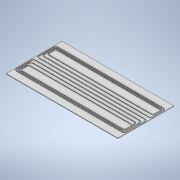
# Autodesk Inventor part: wire_holder_lasercutting800
Saved by Autodesk Inventor 2021 (Build 250183000, 183)
## iProperties
Created: 2021-02-03
Part Number: wire_holder_lasercutting800
Material: Generic
Document SubType Name: Modeling
Designer: User
Density: 1 g/cm^3
Appearance: Default
Author: User
Autodesk Inventor part; units mm, degrees
ref_plane "YZ Plane" through (0, 0, 0) normal (1, 0, 0) x (0, 1, 0)
ref_plane "XZ Plane" through (0, 0, 0) normal (0, 1, 0) x (-1, 0, 0)
ref_plane "XY Plane" through (0, 0, 0) normal (0, 0, 1) x (1, 0, 0)
sketch "Sketch1" plane through (0, 0, 0) normal (0, 1, 0) x (-1, 0, 0)
  line L0 (-18.4221, -16) -> (-503.4221, -16)
  line L1 (-518.4221, -1) -> (-518.4221, 135)
  line L2 (-503.4221, 150) -> (256.5779, 150)
  line L3 (271.5779, 135) -> (271.5779, 26)
  line L4 (-18.4221, -11) -> (-503.4221, -11)
  line L5 (-513.4221, -1) -> (-513.4221, 135)
  line L6 (-503.4221, 145) -> (256.5779, 145)
  line L7 (266.5779, 135) -> (266.5779, 26)
  line L8 (256.5779, 16) -> (-493.4221, 16)
  line L9 (-503.4221, 26) -> (-503.4221, 125)
  line L10 (256.5779, 11) -> (-493.4221, 11)
  line L11 (-508.4221, 26) -> (-508.4221, 125)
  line L12 (-493.4221, 135) -> (246.5779, 135)
  line L13 (-493.4221, 140) -> (246.5779, 140)
  line L14 (256.5779, 125) -> (256.5779, 53)
  line L15 (246.5779, 43) -> (-483.4221, 43)
  line L16 (261.5779, 125) -> (261.5779, 53)
  line L17 (246.5779, 38) -> (-483.4221, 38)
  line L18 (-493.4221, 53) -> (-493.4221, 115)
  line L19 (-483.4221, 125) -> (236.5779, 125)
  line L20 (246.5779, 115) -> (246.5779, 80)
  line L21 (236.5779, 70) -> (-488.4221, 70)
  line L22 (-498.4221, 53) -> (-498.4221, 115)
  line L23 (-483.4221, 130) -> (236.5779, 130)
  line L24 (251.5779, 115) -> (251.5779, 80)
  line L25 (236.5779, 65) -> (-488.4221, 65)
  line L26 (-488.4221, 70) -> (-488.4221, 65)
  line L27 (-123.4221, 150) -> (-123.4221, -150) construction
  line L28 (-18.4221, -11) -> (256.5779, -11)
  line L29 (271.5779, -26) -> (271.5779, -135)
  line L30 (256.5779, -150) -> (-503.4221, -150)
  line L31 (-518.4221, -135) -> (-518.4221, -53)
  line L32 (-18.4221, -16) -> (256.5779, -16)
  line L33 (266.5779, -26) -> (266.5779, -135)
  line L34 (256.5779, -145) -> (-503.4221, -145)
  line L35 (-503.4221, -38) -> (246.5779, -38)
  line L36 (261.5779, -53) -> (261.5779, -125)
  line L37 (246.5779, -140) -> (-493.4221, -140)
  line L38 (-513.4221, -135) -> (-513.4221, -53)
  line L39 (-503.4221, -43) -> (246.5779, -43)
  line L40 (256.5779, -53) -> (256.5779, -125)
  line L41 (246.5779, -135) -> (-493.4221, -135)
  line L42 (-503.4221, -125) -> (-503.4221, -80)
  line L43 (-508.4221, -125) -> (-508.4221, -80)
  line L44 (-493.4221, -65) -> (236.5779, -65)
  line L45 (251.5779, -80) -> (251.5779, -115)
  line L46 (-493.4221, -70) -> (236.5779, -70)
  line L47 (246.5779, -80) -> (246.5779, -115)
  line L48 (236.5779, -125) -> (-498.4221, -125)
  line L49 (236.5779, -130) -> (-498.4221, -130)
  line L50 (-498.4221, -130) -> (-498.4221, -125)
  line L51 (276.5779, 200) -> (276.5779, -200)
  line L52 (276.5779, -200) -> (-523.4221, -200)
  line L53 (-523.4221, -200) -> (-523.4221, 200)
  line L54 (-523.4221, 200) -> (276.5779, 200)
  line L55 (276.5779, 200) -> (276.5779, -200)
  arc A0 (256.5779, -145) -> (266.5779, -135) centre (256.5779, -135) ccw
  arc A1 (256.5779, -150) -> (271.5779, -135) centre (256.5779, -135) ccw
  arc A2 (246.5779, -140) -> (261.5779, -125) centre (246.5779, -125) ccw
  arc A3 (246.5779, -135) -> (256.5779, -125) centre (246.5779, -125) ccw
  arc A4 (236.5779, -125) -> (246.5779, -115) centre (236.5779, -115) ccw
  arc A5 (236.5779, -130) -> (251.5779, -115) centre (236.5779, -115) ccw
  arc A6 (246.5779, -80) -> (236.5779, -70) centre (236.5779, -80) ccw
  arc A7 (251.5779, -80) -> (236.5779, -65) centre (236.5779, -80) ccw
  arc A8 (261.5779, -53) -> (246.5779, -38) centre (246.5779, -53) ccw
  arc A9 (256.5779, -53) -> (246.5779, -43) centre (246.5779, -53) ccw
  arc A10 (266.5779, -26) -> (256.5779, -16) centre (256.5779, -26) ccw
  arc A11 (271.5779, -26) -> (256.5779, -11) centre (256.5779, -26) ccw
  arc A12 (256.5779, 11) -> (271.5779, 26) centre (256.5779, 26) ccw
  arc A13 (256.5779, 16) -> (266.5779, 26) centre (256.5779, 26) ccw
  arc A14 (266.5779, 135) -> (256.5779, 145) centre (256.5779, 135) ccw
  arc A15 (271.5779, 135) -> (256.5779, 150) centre (256.5779, 135) ccw
  arc A16 (261.5779, 125) -> (246.5779, 140) centre (246.5779, 125) ccw
  arc A17 (256.5779, 125) -> (246.5779, 135) centre (246.5779, 125) ccw
  arc A18 (246.5779, 115) -> (236.5779, 125) centre (236.5779, 115) ccw
  arc A19 (251.5779, 115) -> (236.5779, 130) centre (236.5779, 115) ccw
  arc A20 (236.5779, 65) -> (251.5779, 80) centre (236.5779, 80) ccw
  arc A21 (246.5779, 38) -> (261.5779, 53) centre (246.5779, 53) ccw
  arc A22 (246.5779, 43) -> (256.5779, 53) centre (246.5779, 53) ccw
  arc A23 (236.5779, 70) -> (246.5779, 80) centre (236.5779, 80) ccw
  arc A24 (-513.4221, -135) -> (-503.4221, -145) centre (-503.4221, -135) ccw
  arc A25 (-503.4221, -125) -> (-493.4221, -135) centre (-493.4221, -125) ccw
  arc A26 (-508.4221, -125) -> (-493.4221, -140) centre (-493.4221, -125) ccw
  arc A27 (-518.4221, -135) -> (-503.4221, -150) centre (-503.4221, -135) ccw
  arc A28 (-493.4221, -65) -> (-508.4221, -80) centre (-493.4221, -80) ccw
  arc A29 (-493.4221, -70) -> (-503.4221, -80) centre (-493.4221, -80) ccw
  arc A30 (-503.4221, -43) -> (-513.4221, -53) centre (-503.4221, -53) ccw
  arc A31 (-503.4221, -38) -> (-518.4221, -53) centre (-503.4221, -53) ccw
  arc A32 (-518.4221, -1) -> (-503.4221, -16) centre (-503.4221, -1) ccw
  arc A33 (-503.4221, 150) -> (-518.4221, 135) centre (-503.4221, 135) ccw
  arc A34 (-513.4221, -1) -> (-503.4221, -11) centre (-503.4221, -1) ccw
  arc A35 (-503.4221, 145) -> (-513.4221, 135) centre (-503.4221, 135) ccw
  arc A36 (-493.4221, 135) -> (-503.4221, 125) centre (-493.4221, 125) ccw
  arc A37 (-483.4221, 125) -> (-493.4221, 115) centre (-483.4221, 115) ccw
  arc A38 (-483.4221, 130) -> (-498.4221, 115) centre (-483.4221, 115) ccw
  arc A39 (-493.4221, 140) -> (-508.4221, 125) centre (-493.4221, 125) ccw
  arc A40 (-508.4221, 26) -> (-493.4221, 11) centre (-493.4221, 26) ccw
  arc A41 (-503.4221, 26) -> (-493.4221, 16) centre (-493.4221, 26) ccw
  arc A42 (-493.4221, 53) -> (-483.4221, 43) centre (-483.4221, 53) ccw
  arc A43 (-498.4221, 53) -> (-483.4221, 38) centre (-483.4221, 53) ccw
  point P0 (-228.4221, 0)
  dimension "d2" = 5
  dimension "d3" = 5
  dimension "d4" = 5
  dimension "d5" = 5
  dimension "d6" = 5
  dimension "d7" = 5
  dimension "d8" = 5
  dimension "d9" = 5
  dimension "d10" = 5
  dimension "d11" = 790
  dimension "d12" = 22
  dimension "d13" = 5
  dimension "d14" = 5
  dimension "d15" = 22
  dimension "d16" = 5
  dimension "d17" = 5
  dimension "d18" = 5
  dimension "d19" = 5
  dimension "d20" = 22
  dimension "d21" = 5
  dimension "d22" = 5
  dimension "d23" = 5
  dimension "d24" = 5
  dimension "d30" = 5
  dimension "d31" = 5
  dimension "d32" = 5
  dimension "d33" = 790
  dimension "d34" = 500
  dimension "d35" = 5
  dimension "d36" = 5
  dimension "d37" = 5
  dimension "d38" = 5
  dimension "d39" = 22
  dimension "d40" = 5
  dimension "d41" = 5
  dimension "d42" = 5
  dimension "d43" = 5
  dimension "d44" = 5
  dimension "d45" = 5
  dimension "d46" = 22
  dimension "d47" = 5
  dimension "d48" = 5
  dimension "d49" = 5
  dimension "d50" = 5
  dimension "d63" = 400
  dimension "d64" = 50
  dimension "d65" = 5
  dimension "d68" = 5
  dimension "d69" = 10
  dimension "d70" = 15
  dimension "d71" = 10
  dimension "d72" = 10
  dimension "d73" = 15
  dimension "d74" = 10
  dimension "d75" = 15
  dimension "d76" = 15
  dimension "d77" = 10
  constraints: 112 end point, 88 point on circle, 88 tangent, 44 centre point, 35 equal radius, 31 perpendicular, 9 horizontal, 8 parallel, 6 vertical, 1 midpoint
  measures "d2" distance between parallel lines of L1 L5
  measures "d3" distance between parallel lines of L2 L6
  measures "d4" distance between parallel lines of L7 L3
  measures "d5" distance between parallel lines of L13 L6
  measures "d6" distance between parallel lines of L5 L11
  measures "d7" distance between parallel lines of L10 L8
  measures "d8" distance between parallel lines of L14 L16
  measures "d9" distance between parallel lines of L13 L12
  measures "d10" distance between parallel lines of L16 L7
  measures "d11" distance between parallel lines of L1 L3
  measures "d12" distance between parallel lines of L4 L10
  measures "d13" distance between parallel lines of L11 L9
  measures "d14" distance between parallel lines of L17 L15
  measures "d15" distance between parallel lines of L8 L17
  measures "d16" distance between parallel lines of L12 L23
  measures "d17" distance between parallel lines of L9 L22
  measures "d18" distance between parallel lines of L23 L19
  measures "d19" distance between parallel lines of L24 L14
  measures "d20" distance between parallel lines of L15 L25
  measures "d21" distance between parallel lines of L24 L20
  measures "d22" distance between parallel lines of L25 L21
  measures "d23" distance between parallel lines of L22 L18
  measures "d24" distance between parallel lines of L18 L26
  measures "d30" distance between parallel lines of L32 L28
  measures "d31" distance between parallel lines of L33 L29
  measures "d32" distance between parallel lines of L30 L34
  measures "d33" distance between parallel lines of L31 L29
  measures "d34" distance from line of point (-228.422, 0) L29
  measures "d35" distance between parallel lines of L31 L38
  measures "d36" distance between parallel lines of L40 L36
  measures "d37" distance between parallel lines of L36 L33
  measures "d38" distance between parallel lines of L35 L39
  measures "d39" distance between parallel lines of L35 L32
  measures "d40" distance between parallel lines of L37 L41
  measures "d41" distance between parallel lines of L34 L37
  measures "d42" distance between parallel lines of L43 L42
  measures "d43" distance between parallel lines of L44 L46
  measures "d44" distance between parallel lines of L47 L45
  measures "d45" distance between parallel lines of L45 L40
  measures "d46" distance between parallel lines of L44 L39
  measures "d47" distance between parallel lines of L38 L43
  measures "d48" distance between parallel lines of L49 L48
  measures "d49" distance between parallel lines of L41 L49
  measures "d50" distance between parallel lines of L42 L50
  measures "d63" distance of L51.start L51.end
  measures "d64" distance between parallel lines of L52 L30
  measures "d65" distance between parallel lines of L51 L29
  measures "d68" distance between parallel lines of L53 L31
  measures "d69" radius of A0
  measures "d70" radius of A1
  measures "d71" radius of A3
  measures "d72" radius of A6
  measures "d73" radius of A7
  measures "d74" radius of A24
  measures "d75" radius of A26
  measures "d76" radius of A40
  measures "d77" radius of A41
extrude "Extrusion1" add sketch "Sketch1" along normal blind 4.5
equation "\"d2\" = d25"
equation "\"d3\" = d25"
equation "\"d4\" = d25"
equation "\"d5\" = d26"
equation "\"d6\" = d26"
equation "\"d7\" = d25"
equation "\"d8\" = d25"
equation "\"d9\" = d25"
equation "\"d10\" = d26"
equation "\"d12\" = d28"
equation "\"d13\" = d25"
equation "\"d14\" = d25"
equation "\"d15\" = d28"
equation "\"d16\" = d26"
equation "\"d17\" = d26"
equation "\"d18\" = d25"
equation "\"d19\" = d25"
equation "\"d20\" = d28"
equation "\"d21\" = d25"
equation "\"d22\" = d25"
equation "\"d23\" = d25"
equation "\"d24\" = d26"
equation "\"d30\" = d51"
equation "\"d31\" = d51"
equation "\"d32\" = d51"
equation "\"d34\" = 0.5 * d52"
equation "\"d35\" = d51"
equation "\"d36\" = d51"
equation "\"d37\" = d53"
equation "\"d38\" = d51"
equation "\"d39\" = d54"
equation "\"d40\" = d51"
equation "\"d41\" = d53"
equation "\"d42\" = d51"
equation "\"d43\" = d51"
equation "\"d44\" = d51"
equation "\"d45\" = d53"
equation "\"d46\" = d54"
equation "\"d47\" = d53"
equation "\"d48\" = d51"
equation "\"d49\" = d53"
equation "\"d50\" = d53"
equation "\"d25\" = 5"
equation "\"d26\" = 5"
equation "\"d28\" = -1.2 * d25 + 0.2 * d29"
equation "\"d51\" = 5"
equation "\"d53\" = 5"
equation "\"d54\" = -1.2 * d51 + 0.2 * d55"
equation "\"d29\" = 140"
equation "\"d55\" = 140"
equation "\"d52\" = 1000"
body "Solid1"
